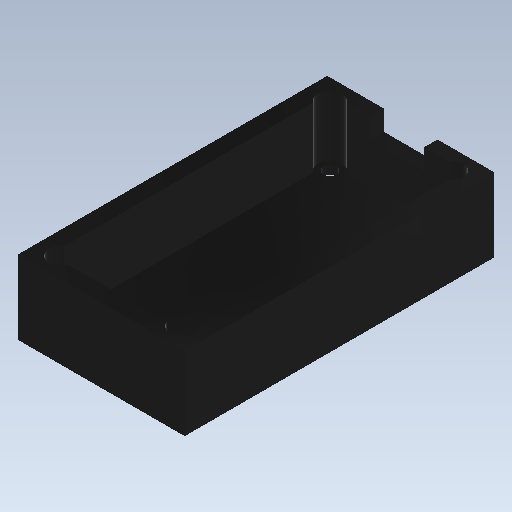
# Autodesk Inventor part: Крышка корпуса задняя
Saved by Autodesk Inventor 2020 (Build 240168000, 168)
## iProperties
Created: 2018-08-28
Part Number: Крышка корпуса задняя
Material: Пластик ПК/АБС
Document SubType Name: Modeling
Designer: Shepelev
Density: 0.357273 g/cm^3
Appearance: Гладкая - черная
Author: Shepelev
Autodesk Inventor part; units mm, degrees
ref_plane "YZ Plane" through (0, 0, 0) normal (1, 0, 0) x (0, 1, 0)
ref_plane "XZ Plane" through (0, 0, 0) normal (0, 1, 0) x (-1, 0, 0)
ref_plane "XY Plane" through (0, 0, 0) normal (0, 0, 1) x (1, 0, 0)
sketch "Эскиз1" plane through (0, 0, 0) normal (0, 1, 0) x (-1, 0, 0)
  line L0 (6.2, 11.5) -> (-6.2, 11.5)
  line L1 (-6.2, 11.5) -> (-6.2, -11.5)
  line L2 (-6.2, -11.5) -> (6.2, -11.5)
  line L3 (6.2, -11.5) -> (6.2, 11.5)
  line L4 (6.2, 11.5) -> (-6.2, -11.5) construction
  line L5 (-6.2, 11.5) -> (6.2, -11.5) construction
  point P0 (0, 0)
  dimension "d0" = 12.4
  dimension "d1" = 23
  constraints: 12 end point, 2 midpoint, 2 parallel, 1 horizontal, 1 perpendicular
  measures "d0" distance of L1.end L2.end
  measures "d1" distance of L0.end L1.end
extrude "Выдавливание1" add sketch "Эскиз1" against normal blind 5.5
sketch "Эскиз2" plane through (0, 0, 0) normal (0, 1, 0) x (1, 0, 0)
  line L0 (-6.2, -11.5) -> (6.2, -11.5) projected
  line L1 (6.2, -11.5) -> (6.2, 11.5) projected
  line L2 (6.2, 11.5) -> (-6.2, 11.5) projected
  line L3 (-6.2, 11.5) -> (-6.2, -11.5) projected
  line L4 (-5, 10.5) -> (5, 10.5)
  line L5 (5, 10.5) -> (5, -10.3)
  line L6 (5, -10.3) -> (-5, -10.3)
  line L7 (-5, -10.3) -> (-5, 10.5)
  line L8 (0, 16.1) -> (0, -16.1) projected
  line L9 (-8.68, 0) -> (8.68, 0) projected
  point P0 (0, 0)
  dimension "d4" = 1
  dimension "d5" = 1.2
  constraints: 8 end point, 2 other
  measures "d4" distance between parallel lines of L2 L4
  measures "d5" distance between parallel lines of L1 L5
extrude "Выдавливание2" cut sketch "Эскиз2" against normal blind 4.5 contours L8 L9 L5 L6 | L6 L7 L9 L8 | L7 L4 L8 L9 | L8 L4 L5 L9
sketch "Эскиз3" plane through (0, 0, 0) normal (0, 1, 0) x (1, 0, 0)
  line L0 (-4.5, -10) -> (4.5, -10)
  line L1 (4.5, -10) -> (4.5, 10)
  line L2 (4.5, 10) -> (-4.5, 10)
  line L3 (-4.5, 10) -> (-4.5, -10)
  line L4 (-4.5, -10) -> (4.5, 10) construction
  line L5 (4.5, -10) -> (-4.5, 10) construction
  point P0 (0, 0)
  dimension "d8" = 9
  dimension "d9" = 20
  constraints: 12 end point, 2 equal length, 2 midpoint, 1 parallel, 1 vertical
  measures "d8" distance of L1.end L2.end
  measures "d9" distance of L0.end L1.end
hole "Отверстие1" at (-4.5, 0, -10) at (4.5, 0, -10) at (4.5, 0, 10) at (-4.5, 0, 10) direction (0, -1, 0) diameter 1 depth 8 tip angle 118 counterbore diameter 1.8 counterbore depth 4.5
sketch "Эскиз4" plane through (0, -5.5, 0) normal (0, -1, 0) x (1, 0, 0)
  circle A0 centre (-4.5, 10) radius 0.5 projected
  circle A1 centre (4.5, 10) radius 0.5 projected
  circle A2 centre (4.5, -10) radius 0.5 projected
  circle A3 centre (-4.5, -10) radius 0.5 projected
  circle A4 centre (-4.5, 10) radius 1
  circle A5 centre (4.5, 10) radius 1
  circle A6 centre (4.5, -10) radius 1
  circle A7 centre (-4.5, -10) radius 1
  point P0 (0, 0)
  dimension "d17" = 2
  constraints: 4 centre point, 3 equal radius
  measures "d17" diameter of A4
extrude "Выдавливание3" cut sketch "Эскиз4" against normal blind 0.5
sketch "Эскиз5" plane through (0, 0, 0) normal (0, 1, 0) x (1, 0, 0)
  line L0 (-2, 10.5) -> (2, 10.5)
  line L1 (2, 10.5) -> (2, 11.5)
  line L2 (2, 11.5) -> (-2, 11.5)
  line L3 (-2, 11.5) -> (-2, 10.5)
  arc A0 (3.6515, -10.3) -> (5, -9.2517) centre (4.5, -10) ccw projected
  line L4 (3.6515, -10.3) -> (-3.6515, -10.3) projected
  arc A1 (-5, -9.2517) -> (-3.6515, -10.3) centre (-4.5, -10) ccw projected
  line L5 (-5, -9.2517) -> (-5, 9.2517) projected
  arc A2 (-3.7517, 10.5) -> (-5, 9.2517) centre (-4.5, 10) ccw projected
  line L6 (-3.7517, 10.5) -> (3.7517, 10.5) projected
  arc A3 (5, 9.2517) -> (3.7517, 10.5) centre (4.5, 10) ccw projected
  line L7 (5, 9.2517) -> (5, -9.2517) projected
  line L8 (-6.2, -11.5) -> (6.2, -11.5) projected
  line L9 (6.2, -11.5) -> (6.2, 11.5) projected
  line L10 (6.2, 11.5) -> (-6.2, 11.5) projected
  line L11 (-6.2, 11.5) -> (-6.2, -11.5) projected
  line L12 (0, 16.1) -> (0, -16.1) projected
  point P0 (0, 0)
  point P1 (0, 11.5)
  point P2 (0, 10.5)
  dimension "d23" = 4
  constraints: 8 end point, 4 midpoint, 2 parallel, 1 horizontal, 1 perpendicular, 1 other
  measures "d23" distance of L0.start L0.end
extrude "Выдавливание4" cut sketch "Эскиз5" against normal blind 1.5 contours L3 L2 L12 L0 | L12 L2 L1 L0
